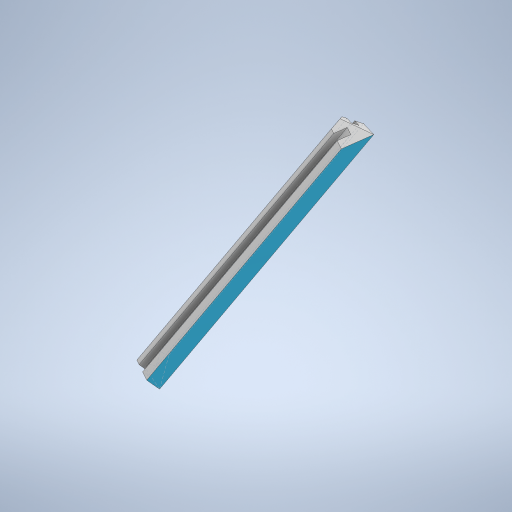
# Autodesk Inventor part: Perfil
Saved by Autodesk Inventor 2024 (Build 280153000, 153)
## iProperties
Created: 2023-07-27
Part Number: Perfil
Material: Genérico
Document SubType Name: Modeling
Designer: sergi
Density: 1 g/cm^3
Appearance: Valor por defecto
Author: sergi
Autodesk Inventor part; units mm, degrees
ref_plane "YZ Plane" through (0, 0, 0) normal (1, 0, 0) x (0, 1, 0)
ref_plane "XZ Plane" through (0, 0, 0) normal (0, 1, 0) x (-1, 0, 0)
ref_plane "XY Plane" through (0, 0, 0) normal (0, 0, 1) x (1, 0, 0)
sketch "Boceto1" plane through (0, 0, 0) normal (0, 1, 0) x (-1, 0, 0)
  line L0 (47.5, 65.3781) -> (76.8566, -24.9722)
  line L1 (76.8566, -24.9722) -> (0, -80.8118)
  line L2 (0, -80.8118) -> (-76.8566, -24.9722)
  line L3 (-76.8566, -24.9722) -> (-47.5, 65.3781)
  line L4 (-47.5, 65.3781) -> (47.5, 65.3781)
  line L5 (0, 0) -> (130.7563, 0) construction
  line L6 (130.7563, 0) -> (130.7563, 130.7563) construction
  line L7 (130.7563, 130.7563) -> (0, 130.7563) construction
  line L8 (0, 130.7563) -> (0, 0) construction
  line L9 (130.7563, 130.7563) -> (0, 65.3781)
  dimension "d0" = 95
  dimension "d1" = 211.5681
  dimension "d2" = 26.565
  constraints: 20 end point, 2 horizontal, 2 midpoint, 2 parallel, 2 perpendicular, 1 coincident, 11 other
  measures "d0" distance of L3.end L0.start
  measures "d1" distance from line of L1.end L7
  measures "d2" angle of L4 L9
extrude "Extrusión1" add sketch "Boceto1" along normal blind 211.5681 draft 26.565
sketch "Boceto2" plane through (0, 211.5681, 0) normal (0, 1, 0) x (1, 0, 0)
  line L0 (0, -80.8118) -> (-76.8566, -24.9722)
  line L1 (-76.8566, -24.9722) -> (-47.5, 65.3781)
  line L2 (-47.5, 65.3781) -> (47.5, 65.3781)
  line L3 (47.5, 65.3781) -> (76.8566, -24.9722)
  line L4 (76.8566, -24.9722) -> (0, -80.8118)
  point P0 (0, 0)
  point P1 (0, 0)
  dimension "L" = 95
  constraints: 10 end point, 1 coincident, 1 horizontal, 11 other
  measures "L" distance of L1.end L2.end
extrude "Extrusión2" cut sketch "Boceto2" against normal blind 211.5681 draft 26.565 keep common part
sketch "Boceto3" plane through (47.5, 0, 65.3781) normal (0.8506508, -0.4472136, 0.2763932) x (0.309017, 0, -0.9510565)
  line L0 (47.5, 146.19) -> (124.3566, 90.3504) projected
  line L1 (-29.3566, 90.3504) -> (47.5, 146.19) projected
  line L2 (0, 0) -> (-29.3566, 90.3504) projected
  line L3 (0, 0) -> (95, 0) projected
  line L4 (95, 0) -> (124.3566, 90.3504) projected
  line L5 (117.3032, 88.0586) -> (47.5, 138.7736)
  line L6 (47.5, 138.7736) -> (-22.3032, 88.0586)
  line L7 (-22.3032, 88.0586) -> (4.3593, 6)
  line L8 (4.3593, 6) -> (90.6407, 6)
  line L9 (90.6407, 6) -> (117.3032, 88.0586)
  point P0 (47.5, -29.238)
  dimension "D" = 6
  constraints: 10 end point, 4 other
  measures "D" distance between parallel lines of L4 L9
extrude "Extrusión3" cut sketch "Boceto3" against normal blind 111.5681 contours L9 L8 L7 L6 L5
sketch "Boceto4" plane through (76.8566, 0, -24.9722) normal (0.5257311, -0.4472136, -0.7236068) x (-0.809017, 0, -0.5877853)
  line L0 (47.5, 146.19) -> (124.3566, 90.3504) projected
  line L1 (-29.3566, 90.3504) -> (47.5, 146.19) projected
  line L2 (0, 0) -> (-29.3566, 90.3504) projected
  line L3 (0, 0) -> (95, 0) projected
  line L4 (95, 0) -> (124.3566, 90.3504) projected
  line L5 (90.6407, 6) -> (4.3593, 6)
  line L6 (4.3593, 6) -> (-22.3032, 88.0586)
  line L7 (-22.3032, 88.0586) -> (47.5, 138.7736)
  line L8 (47.5, 138.7736) -> (117.3032, 88.0586)
  line L9 (117.3032, 88.0586) -> (90.6407, 6)
  point P0 (47.5, -29.238)
  dimension "d14" = 6
  constraints: 10 end point, 4 other
  measures "d14" distance between parallel lines of L3 L5
extrude "Extrusión4" cut sketch "Boceto4" against normal blind 111.5681 contours L5 L6 L7 L8 L9
sketch "Boceto5" plane through (0, 0, 0) normal (0, -1, 0) x (1, 0, 0)
  line L0 (76.8566, -24.9722) -> (0, -80.8118) projected
  line L1 (47.5, 65.3781) -> (76.8566, -24.9722) projected
  line L2 (-47.5, 65.3781) -> (47.5, 65.3781) projected
  line L3 (-76.8566, -24.9722) -> (-47.5, 65.3781) projected
  line L4 (0, -80.8118) -> (-76.8566, -24.9722) projected
  line L5 (43.1407, 59.3781) -> (69.8032, -22.6804)
  line L6 (69.8032, -22.6804) -> (0, -73.3954)
  line L7 (0, -73.3954) -> (-69.8032, -22.6804)
  line L8 (-69.8032, -22.6804) -> (-43.1407, 59.3781)
  line L9 (-43.1407, 59.3781) -> (43.1407, 59.3781)
  point P0 (0, 0)
  dimension "d17" = 6
  constraints: 10 end point, 4 other
  measures "d17" distance between parallel lines of L2 L9
extrude "Extrusión5" cut sketch "Boceto5" against normal blind 111.5681 contours L5 L6 L7 L8 L9
sketch "Boceto6" plane through (47.5, 211.5681, -65.3781) normal (0, 0.4472136, -0.8944272) x (-1, 0, 0)
  line L0 (47.5, -146.19) -> (124.3566, -90.3504) projected
  line L1 (95, 0) -> (124.3566, -90.3504) projected
  line L2 (95, 0) -> (0, 0) projected
  line L3 (0, 0) -> (-29.3566, -90.3504) projected
  line L4 (-29.3566, -90.3504) -> (47.5, -146.19) projected
  line L5 (117.3032, -88.0586) -> (47.5, -138.7736)
  line L6 (47.5, -138.7736) -> (-22.3032, -88.0586)
  line L7 (-22.3032, -88.0586) -> (4.3593, -6)
  line L8 (4.3593, -6) -> (90.6407, -6)
  line L9 (90.6407, -6) -> (117.3032, -88.0586)
  point P0 (47.5, -159.9943)
  dimension "d20" = 6
  constraints: 10 end point, 4 other
  measures "d20" distance between parallel lines of L0 L5
extrude "Extrusión6" cut sketch "Boceto6" against normal blind 111.5681 contours L5 L6 L7 L8 L9
sketch "Boceto7" plane through (0, 0, -80.8118) normal (-0.5257311, -0.4472136, -0.7236068) x (-0.809017, 0, 0.5877853)
  line L0 (47.5, 146.19) -> (124.3566, 90.3504) projected
  line L1 (-29.3566, 90.3504) -> (47.5, 146.19) projected
  line L2 (0, 0) -> (-29.3566, 90.3504) projected
  line L3 (0, 0) -> (95, 0) projected
  line L4 (95, 0) -> (124.3566, 90.3504) projected
  line L5 (117.3032, 88.0586) -> (47.5, 138.7736)
  line L6 (47.5, 138.7736) -> (-22.3032, 88.0586)
  line L7 (-22.3032, 88.0586) -> (4.3593, 6)
  line L8 (4.3593, 6) -> (90.6407, 6)
  line L9 (90.6407, 6) -> (117.3032, 88.0586)
  point P0 (47.5, -29.238)
  dimension "d23" = 6
  constraints: 10 end point, 4 other
  measures "d23" distance between parallel lines of L4 L9
extrude "Extrusión7" cut sketch "Boceto7" against normal blind 111.5681 contours L9 L8 L7 L6 L5
sketch "Boceto8" plane through (76.8566, 211.5681, 24.9722) normal (0.8506508, 0.4472136, -0.2763932) x (-0.309017, 0, -0.9510565)
  line L0 (47.5, -146.19) -> (124.3566, -90.3504) projected
  line L1 (95, 0) -> (124.3566, -90.3504) projected
  line L2 (95, 0) -> (0, 0) projected
  line L3 (0, 0) -> (-29.3566, -90.3504) projected
  line L4 (-29.3566, -90.3504) -> (47.5, -146.19) projected
  line L5 (47.5, -138.7736) -> (117.3032, -88.0586)
  line L6 (117.3032, -88.0586) -> (90.6407, -6)
  line L7 (90.6407, -6) -> (4.3593, -6)
  line L8 (4.3593, -6) -> (-22.3032, -88.0586)
  line L9 (-22.3032, -88.0586) -> (47.5, -138.7736)
  point P0 (47.5, -159.9943)
  dimension "d26" = 6
  constraints: 10 end point, 4 other
  measures "d26" distance between parallel lines of L4 L9
extrude "Extrusión8" cut sketch "Boceto8" against normal blind 111.5681 contours L9 L8 L7 L6 L5
sketch "Boceto9" plane through (0, 211.5681, 0) normal (0, 1, 0) x (1, 0, 0)
  line L0 (78.0615, -19.9972) -> (-16.844, -50.8338) projected
  line L1 (-47.5, 65.3781) -> (47.5, 65.3781) projected
  line L2 (-76.8566, -24.9722) -> (-47.5, 65.3781) projected
  line L3 (0, -80.8118) -> (-76.8566, -24.9722) projected
  line L4 (76.8566, -24.9722) -> (0, -80.8118) projected
  line L5 (47.5, 65.3781) -> (76.8566, -24.9722) projected
  line L6 (0, -73.3954) -> (-69.8032, -22.6804)
  line L7 (-69.8032, -22.6804) -> (-43.1407, 59.3781)
  line L8 (-43.1407, 59.3781) -> (43.1407, 59.3781)
  line L9 (43.1407, 59.3781) -> (69.8032, -22.6804)
  line L10 (69.8032, -22.6804) -> (0, -73.3954)
  point P0 (0, 0)
  dimension "d29" = 6
  constraints: 10 end point, 4 other
  measures "d29" distance between parallel lines of L4 L10
extrude "Extrusión9" cut sketch "Boceto9" against normal blind 111.5681 contours L6 L7 L8 L9 L10
sketch "Boceto10" plane through (-47.5, 211.5681, -65.3781) normal (-0.8506508, 0.4472136, -0.2763932) x (-0.309017, 0, 0.9510565)
  line L0 (-29.3566, -90.3504) -> (47.5, -146.19) projected
  line L1 (47.5, -146.19) -> (124.3566, -90.3504) projected
  line L2 (95, 0) -> (124.3566, -90.3504) projected
  line L3 (95, 0) -> (0, 0) projected
  line L4 (0, 0) -> (-29.3566, -90.3504) projected
  line L5 (117.3032, -88.0586) -> (47.5, -138.7736)
  line L6 (47.5, -138.7736) -> (-22.3032, -88.0586)
  line L7 (-22.3032, -88.0586) -> (4.3593, -6)
  line L8 (4.3593, -6) -> (90.6407, -6)
  line L9 (90.6407, -6) -> (117.3032, -88.0586)
  point P0 (47.5, -159.9943)
  dimension "d32" = 6
  constraints: 10 end point, 4 other
  measures "d32" distance between parallel lines of L2 L9
extrude "Extrusión10" cut sketch "Boceto10" against normal blind 111.5681 contours L5 L6 L7 L8 L9
sketch "Boceto11" plane through (-76.8566, 0, -24.9722) normal (-0.8506508, -0.4472136, 0.2763932) x (0.309017, 0, 0.9510565)
  line L0 (47.5, 65.3781) -> (90.6407, 79.3954) projected
  line L1 (-29.3566, 90.3504) -> (47.5, 146.19) projected
  line L2 (0, 0) -> (-29.3566, 90.3504) projected
  line L3 (0, 0) -> (95, 0) projected
  line L4 (95, 0) -> (124.3566, 90.3504) projected
  line L5 (47.5, 146.19) -> (124.3566, 90.3504) projected
  line L6 (117.3032, 88.0586) -> (90.6407, 6)
  line L7 (90.6407, 6) -> (4.3593, 6)
  line L8 (4.3593, 6) -> (-22.3032, 88.0586)
  line L9 (-22.3032, 88.0586) -> (47.5, 138.7736)
  line L10 (47.5, 138.7736) -> (117.3032, 88.0586)
  point P0 (47.5, -29.238)
  dimension "d35" = 6
  constraints: 10 end point, 4 other
  measures "d35" distance between parallel lines of L4 L6
extrude "Extrusión11" cut sketch "Boceto11" against normal blind 111.5681 contours L6 L7 L8 L9 L10
sketch "Boceto12" plane through (-47.5, 0, 65.3781) normal (0, -0.4472136, 0.8944272) x (1, 0, 0)
  line L0 (4.3593, 6) -> (47.5, 65.3781) projected
  line L1 (-29.3566, 90.3504) -> (47.5, 146.19) projected
  line L2 (0, 0) -> (-29.3566, 90.3504) projected
  line L3 (0, 0) -> (95, 0) projected
  line L4 (95, 0) -> (124.3566, 90.3504) projected
  line L5 (47.5, 146.19) -> (124.3566, 90.3504) projected
  line L6 (117.3032, 88.0586) -> (90.6407, 6)
  line L7 (90.6407, 6) -> (4.3593, 6)
  line L8 (4.3593, 6) -> (-22.3032, 88.0586)
  line L9 (-22.3032, 88.0586) -> (47.5, 138.7736)
  line L10 (47.5, 138.7736) -> (117.3032, 88.0586)
  point P0 (47.5, -29.238)
  dimension "d38" = 6
  constraints: 10 end point, 4 other
  measures "d38" distance between parallel lines of L5 L10
extrude "Extrusión12" cut sketch "Boceto12" against normal blind 111.5681 contours L6 L7 L8 L9 L10
sketch "Boceto13" plane through (0, 211.5681, 80.8118) normal (0.5257311, 0.4472136, 0.7236068) x (0.809017, 0, -0.5877853)
  line L0 (-29.3566, -90.3504) -> (47.5, -146.19) projected
  line L1 (47.5, -146.19) -> (124.3566, -90.3504) projected
  line L2 (95, 0) -> (124.3566, -90.3504) projected
  line L3 (95, 0) -> (0, 0) projected
  line L4 (0, 0) -> (-29.3566, -90.3504) projected
  line L5 (47.5, -138.7736) -> (-22.3032, -88.0586)
  line L6 (-22.3032, -88.0586) -> (4.3593, -6)
  line L7 (4.3593, -6) -> (90.6407, -6)
  line L8 (90.6407, -6) -> (117.3032, -88.0586)
  line L9 (117.3032, -88.0586) -> (47.5, -138.7736)
  point P0 (47.5, -159.9943)
  dimension "d41" = 6
  constraints: 10 end point, 4 other
  measures "d41" distance between parallel lines of L0 L5
extrude "Extrusión13" cut sketch "Boceto13" against normal blind 111.5681 contours L5 L6 L7 L8 L9
sketch "Boceto14" plane through (-76.8566, 211.5681, 24.9722) normal (-0.5257311, 0.4472136, 0.7236068) x (0.809017, 0, 0.5877853)
  line L0 (-29.3566, -90.3504) -> (47.5, -146.19) projected
  line L1 (47.5, -146.19) -> (124.3566, -90.3504) projected
  line L2 (95, 0) -> (124.3566, -90.3504) projected
  line L3 (95, 0) -> (0, 0) projected
  line L4 (0, 0) -> (-29.3566, -90.3504) projected
  line L5 (-22.3032, -88.0586) -> (47.5, -138.7736)
  line L6 (47.5, -138.7736) -> (117.3032, -88.0586)
  line L7 (117.3032, -88.0586) -> (90.6407, -6)
  line L8 (90.6407, -6) -> (4.3593, -6)
  line L9 (4.3593, -6) -> (-22.3032, -88.0586)
  point P0 (47.5, -159.9943)
  dimension "d44" = 6
  constraints: 10 end point, 4 other
  measures "d44" distance between parallel lines of L4 L9
extrude "Extrusión14" cut sketch "Boceto14" against normal blind 111.5681 contours L9 L8 L7 L6 L5
ref_plane "Plano de trabajo1" through (47.5, 210.2265, -62.6949) normal (0, 0.4472136, -0.8944272) x (-1, 0, 0)
sketch "Boceto15" plane through (47.5, 210.2265, -62.6949) normal (0, 0.4472136, -0.8944272) x (-1, 0, 0)
  line L0 (4.3593, -6) -> (90.6407, -6) projected
  line L1 (-22.3032, -88.0586) -> (4.3593, -6) projected
  line L2 (47.5, -138.7736) -> (-22.3032, -88.0586) projected
  line L3 (117.3032, -88.0586) -> (47.5, -138.7736) projected
  line L4 (90.6407, -6) -> (117.3032, -88.0586) projected
  line L5 (2.5429, -3.5) -> (92.4571, -3.5)
  line L6 (92.4571, -3.5) -> (120.2421, -89.0135)
  line L7 (120.2421, -89.0135) -> (47.5, -141.8637)
  line L8 (47.5, -141.8637) -> (-25.2421, -89.0135)
  line L9 (-25.2421, -89.0135) -> (2.5429, -3.5)
  point P0 (47.5, -159.9943)
  dimension "D2" = 2.5
  constraints: 10 end point, 4 other
  measures "D2" distance between parallel lines of L1 L9
extrude "Extrusión15" cut sketch "Boceto15" along normal mid plane 1.8 contours L0 L4 L3 L2 L1 | L5 L6 L7 L8 L9
ref_plane "Plano de trabajo2" through (75.2794, 1.3416, -22.8014) normal (0.5257311, -0.4472136, -0.7236068) x (-0.809017, 0, -0.5877853)
sketch "Boceto16" plane through (75.2794, 1.3416, -22.8014) normal (0.5257311, -0.4472136, -0.7236068) x (-0.809017, 0, -0.5877853)
  line L0 (90.6407, 6) -> (4.3593, 6) projected
  line L1 (117.3032, 88.0586) -> (90.6407, 6) projected
  line L2 (47.5, 138.7736) -> (117.3032, 88.0586) projected
  line L3 (-22.3032, 88.0586) -> (47.5, 138.7736) projected
  line L4 (4.3593, 6) -> (-22.3032, 88.0586) projected
  line L5 (2.5429, 3.5) -> (92.4571, 3.5)
  line L6 (92.4571, 3.5) -> (120.2421, 89.0135)
  line L7 (120.2421, 89.0135) -> (47.5, 141.8637)
  line L8 (47.5, 141.8637) -> (-25.2421, 89.0135)
  line L9 (-25.2421, 89.0135) -> (2.5429, 3.5)
  point P0 (47.5, -29.238)
  dimension "d52" = 2.5
  constraints: 10 end point, 4 other
  measures "d52" distance between parallel lines of L0 L5
extrude "Extrusión16" cut sketch "Boceto16" along normal mid plane 1.8
ref_plane "Plano de trabajo3" through (74.3047, 210.2265, 25.8014) normal (0.8506508, 0.4472136, -0.2763932) x (-0.309017, 0, -0.9510565)
sketch "Boceto17" plane through (74.3047, 210.2265, 25.8014) normal (0.8506508, 0.4472136, -0.2763932) x (-0.309017, 0, -0.9510565)
  line L0 (47.5, -138.7736) -> (-22.3032, -88.0586) projected
  line L1 (117.3032, -88.0586) -> (47.5, -138.7736) projected
  line L2 (90.6407, -6) -> (117.3032, -88.0586) projected
  line L3 (4.3593, -6) -> (90.6407, -6) projected
  line L4 (-22.3032, -88.0586) -> (4.3593, -6) projected
  line L5 (-25.2421, -89.0135) -> (47.5, -141.8637)
  line L6 (47.5, -141.8637) -> (120.2421, -89.0135)
  line L7 (120.2421, -89.0135) -> (92.4571, -3.5)
  line L8 (92.4571, -3.5) -> (2.5429, -3.5)
  line L9 (2.5429, -3.5) -> (-25.2421, -89.0135)
  point P0 (47.5, -159.9943)
  dimension "d56" = 2.5
  constraints: 10 end point, 4 other
  measures "d56" distance between parallel lines of L0 L5
extrude "Extrusión17" cut sketch "Boceto17" along normal mid plane 1.8
ref_plane "Plano de trabajo4" through (1.5772, 1.3416, -78.641) normal (-0.5257311, -0.4472136, -0.7236068) x (-0.809017, 0, 0.5877853)
sketch "Boceto18" plane through (1.5772, 1.3416, -78.641) normal (-0.5257311, -0.4472136, -0.7236068) x (-0.809017, 0, 0.5877853)
  line L0 (117.3032, 88.0586) -> (90.6407, 6) projected
  line L1 (47.5, 138.7736) -> (117.3032, 88.0586) projected
  line L2 (-22.3032, 88.0586) -> (47.5, 138.7736) projected
  line L3 (4.3593, 6) -> (-22.3032, 88.0586) projected
  line L4 (90.6407, 6) -> (4.3593, 6) projected
  line L5 (92.4571, 3.5) -> (120.2421, 89.0135)
  line L6 (120.2421, 89.0135) -> (47.5, 141.8637)
  line L7 (47.5, 141.8637) -> (-25.2421, 89.0135)
  line L8 (-25.2421, 89.0135) -> (2.5429, 3.5)
  line L9 (2.5429, 3.5) -> (92.4571, 3.5)
  point P0 (47.5, -29.238)
  dimension "d60" = 2.5
  constraints: 10 end point, 4 other
  measures "d60" distance between parallel lines of L0 L5
extrude "Extrusión18" cut sketch "Boceto18" along normal mid plane 1.8 contours L0 L4 L3 L2 L1 | L9 L8 L7 L6 L5
ref_plane "Plano de trabajo5" through (0, 3, 0) normal (0, -1, 0) x (1, 0, 0)
sketch "Boceto19" plane through (0, 3, 0) normal (0, -1, 0) x (1, 0, 0)
  line L0 (0, -73.3954) -> (-69.8032, -22.6804) projected
  line L1 (-69.8032, -22.6804) -> (-43.1407, 59.3781) projected
  line L2 (-43.1407, 59.3781) -> (43.1407, 59.3781) projected
  line L3 (43.1407, 59.3781) -> (69.8032, -22.6804) projected
  line L4 (69.8032, -22.6804) -> (0, -73.3954) projected
  line L5 (76.8566, -24.9722) -> (0, -80.8118) projected
  line L6 (47.5, 65.3781) -> (76.8566, -24.9722) projected
  line L7 (-47.5, 65.3781) -> (47.5, 65.3781) projected
  line L8 (-76.8566, -24.9722) -> (-47.5, 65.3781) projected
  line L9 (0, -80.8118) -> (-76.8566, -24.9722) projected
  line L10 (-44.9571, 61.8781) -> (-72.7421, -23.6353)
  line L11 (-72.7421, -23.6353) -> (0, -76.4856)
  line L12 (0, -76.4856) -> (72.7421, -23.6353)
  line L13 (72.7421, -23.6353) -> (44.9571, 61.8781)
  line L14 (44.9571, 61.8781) -> (-44.9571, 61.8781)
  point P0 (0, 0)
  dimension "d64" = 2.5
  constraints: 10 end point, 4 other
  measures "d64" distance between parallel lines of L1 L10
extrude "Extrusión19" cut sketch "Boceto19" along normal mid plane 1.8 contours L0 L1 L2 L3 L4 | L14 L13 L12 L11 L10
ref_plane "Plano de trabajo6" through (44.948, 1.3416, 64.549) normal (0.8506508, -0.4472136, 0.2763932) x (0.309017, 0, -0.9510565)
sketch "Boceto20" plane through (44.948, 1.3416, 64.549) normal (0.8506508, -0.4472136, 0.2763932) x (0.309017, 0, -0.9510565)
  line L0 (4.3593, 6) -> (-22.3032, 88.0586) projected
  line L1 (-22.3032, 88.0586) -> (47.5, 138.7736) projected
  line L2 (47.5, 138.7736) -> (117.3032, 88.0586) projected
  line L3 (117.3032, 88.0586) -> (90.6407, 6) projected
  line L4 (90.6407, 6) -> (4.3593, 6) projected
  line L5 (47.5, 146.19) -> (124.3566, 90.3504) projected
  line L6 (-29.3566, 90.3504) -> (47.5, 146.19) projected
  line L7 (0, 0) -> (-29.3566, 90.3504) projected
  line L8 (0, 0) -> (95, 0) projected
  line L9 (95, 0) -> (124.3566, 90.3504) projected
  line L10 (-25.2421, 89.0135) -> (2.5429, 3.5)
  line L11 (2.5429, 3.5) -> (92.4571, 3.5)
  line L12 (92.4571, 3.5) -> (120.2421, 89.0135)
  line L13 (120.2421, 89.0135) -> (47.5, 141.8637)
  line L14 (47.5, 141.8637) -> (-25.2421, 89.0135)
  point P0 (47.5, -29.238)
  dimension "d68" = 2.5
  constraints: 10 end point, 4 other
  measures "d68" distance between parallel lines of L0 L10
extrude "Extrusión20" cut sketch "Boceto20" along normal mid plane 1.8 contours L0 L1 L2 L3 L4 | L14 L13 L12 L11 L10
ref_plane "Plano de trabajo7" through (121.2022, 87.4453, -39.381) normal (-0.309017, 0, -0.9510565) x (-0.8506508, -0.4472136, 0.2763932)
split body "Dividir1" result two bodies by plane through (121.2022, 87.4453, -39.381) normal (-0.309017, 0, -0.9510565) first body at (-25.6189, 99.4475, -120.8794)
ref_plane "Plano de trabajo8" through (118.0478, 78.762, -43.7226) normal (0, -0.8506508, 0.5257311) x (-0.5257311, 0.4472136, 0.7236068)
split "Dividir2" plane through (118.0478, 78.762, -43.7226) removes the side toward (0, 0.8506508, -0.5257311) bodies 2
ref_plane "Plano de trabajo9" through (121.2022, 78.762, -34.0144) normal (-0.309017, -0.8506508, -0.4253254) x (-0.8506508, 0.4472136, -0.2763932)
split "Dividir3" plane through (121.2022, 78.762, -34.0144) removes the side toward (0.309017, 0.8506508, 0.4253254) bodies 3
ref_plane "Plano de trabajo13" through (34.9016, 9.7082, -48.0379) normal (-0.5, -0.5257311, 0.688191) x (0.809017, 0, 0.5877853)
split "Dividir7" plane through (34.9016, 9.7082, -48.0379) removes the side toward (-0.5, -0.5257311, 0.688191) bodies 3
ref_plane "Plano de trabajo14" through (74.9071, 5.3666, -29.7054) normal (-0.809017, -0.5257311, -0.2628656) x (-0.5257311, 0.4472136, 0.7236068)
split "Dividir8" plane through (74.9071, 5.3666, -29.7054) removes the side toward (-0.809017, -0.5257311, -0.2628656) bodies 2
ref_plane "Plano de trabajo16" through (107.0671, 64.0042, -31.5775) normal (-0.809017, 0.5257311, 0.2628656) x (0.5, 0.8506508, -0.1624598)
ref_plane "Plano de trabajo15" through (107.8761, 63.4785, -31.8404) normal (-0.809017, 0.5257311, 0.2628656) x (0.5, 0.8506508, -0.1624598)
combine bodies "Combinar1" operation type add bodies to combine 3 2
split "Dividir9" plane through (107.0671, 64.0042, -31.5775) removes the side toward (-0.809017, 0.5257311, 0.2628656) bodies 3
equation "\"d0\" = L"
equation "\"d3\" = d1"
equation "\"d4\" = d2"
equation "\"d6\" = d1"
equation "\"d7\" = d2"
equation "\"d14\" = D"
equation "\"d17\" = D"
equation "\"d20\" = D"
equation "\"d23\" = D"
equation "\"d26\" = D"
equation "\"d29\" = D"
equation "\"d32\" = D"
equation "\"d35\" = D"
equation "\"d38\" = D"
equation "\"d41\" = D"
equation "\"d44\" = D"
equation "\"d48\" = ESP"
equation "\"d52\" = D2"
equation "\"d56\" = D2"
equation "\"d57\" = ESP"
equation "\"d60\" = D2"
equation "\"d61\" = ESP"
equation "\"d64\" = D2"
equation "\"d65\" = ESP"
equation "\"d68\" = D2"
equation "\"d69\" = ESP"
equation "\"d51\" = P"
equation "\"d55\" = P"
equation "\"d59\" = P"
equation "\"d63\" = P"
equation "\"d67\" = P"
equation "\"ESP\" = 1.8"
equation "\"P\" = -3"
